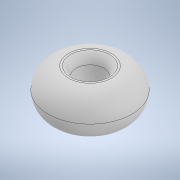
# Autodesk Inventor part: 8001_250uH_DCore_2layer_Tx_Filter_MPSv2_v1
Saved by Autodesk Inventor 2021 (Build 250183000, 183)
## iProperties
Created: 2020-12-10
Part Number: 8001_250uH_DCore_2layer_Tx_Filter_MPSv2_v1
Material: Generic
Document SubType Name: Modeling
Designer: Barksdale
Density: 1 g/cm^3
Appearance: Default
Author: Barksdale
Autodesk Inventor part; units mm, degrees
ref_plane "YZ Plane" through (0, 0, 0) normal (1, 0, 0) x (0, 1, 0)
ref_plane "XZ Plane" through (0, 0, 0) normal (0, 1, 0) x (-1, 0, 0)
ref_plane "XY Plane" through (0, 0, 0) normal (0, 0, 1) x (1, 0, 0)
sketch "Sketch1" plane through (0, 0, 0) normal (0, 0, 1) x (1, 0, 0)
  line L0 (0, 0) -> (12.8, 0)
  line L1 (0, 0) -> (38.35, 0)
  line L2 (0, 0) -> (22.1, 0)
  line L3 (12.8, 0) -> (28.4, 0)
  line L4 (0, 0) -> (22.1, 0)
  line L5 (12.8, 0) -> (12.8, 10.9)
  line L6 (12.8, 0) -> (12.8, -10.9)
  line L7 (0, 0) -> (0, 15.6)
  arc A0 (17.9048, 19.2) -> (12.8, 10.9) centre (22.1, 10.9) ccw
  line L8 (22.1, 18.9374) -> (22.1, 19.2)
  line L9 (19.6691, 19.2) -> (17.9048, 19.2)
  arc A1 (38.35, 0) -> (17.9048, 19.2) centre (18.7869, -0.3462) ccw
  line L10 (12.8, 0) -> (12.8, -10.9)
  arc A2 (12.8, -10.9) -> (17.9048, -19.2) centre (22.1, -10.9) ccw
  arc A3 (17.9048, -19.2) -> (38.35, 0) centre (18.7869, 0.3462) ccw
  dimension "d0" = 12.8
  dimension "d1" = 38.35
  dimension "d4" = 22.1
  dimension "d5" = 10.9
  dimension "d8" = 19.2
  constraints: 22 end point, 10 point on circle, 4 centre point, 4 symmetric about line, 3 point on line, 2 horizontal, 2 perpendicular, 2 vertical, 2 other
  measures "d0" distance of L0.start L0.end
  measures "d1" distance of L0.start L1.end
  measures "d4" distance of L0.start L4.end
  measures "d5" distance of L5.end L0.end
  measures "d8" distance of L4.end L8.end
revolve "Revolution2" add sketch "Sketch1" angle 360 about axis through (0, 0, 0) along (0, 1, 0) contours L5 A0 L9 A1 L1 | L1 A3 A2 L6
body "Solid2"
